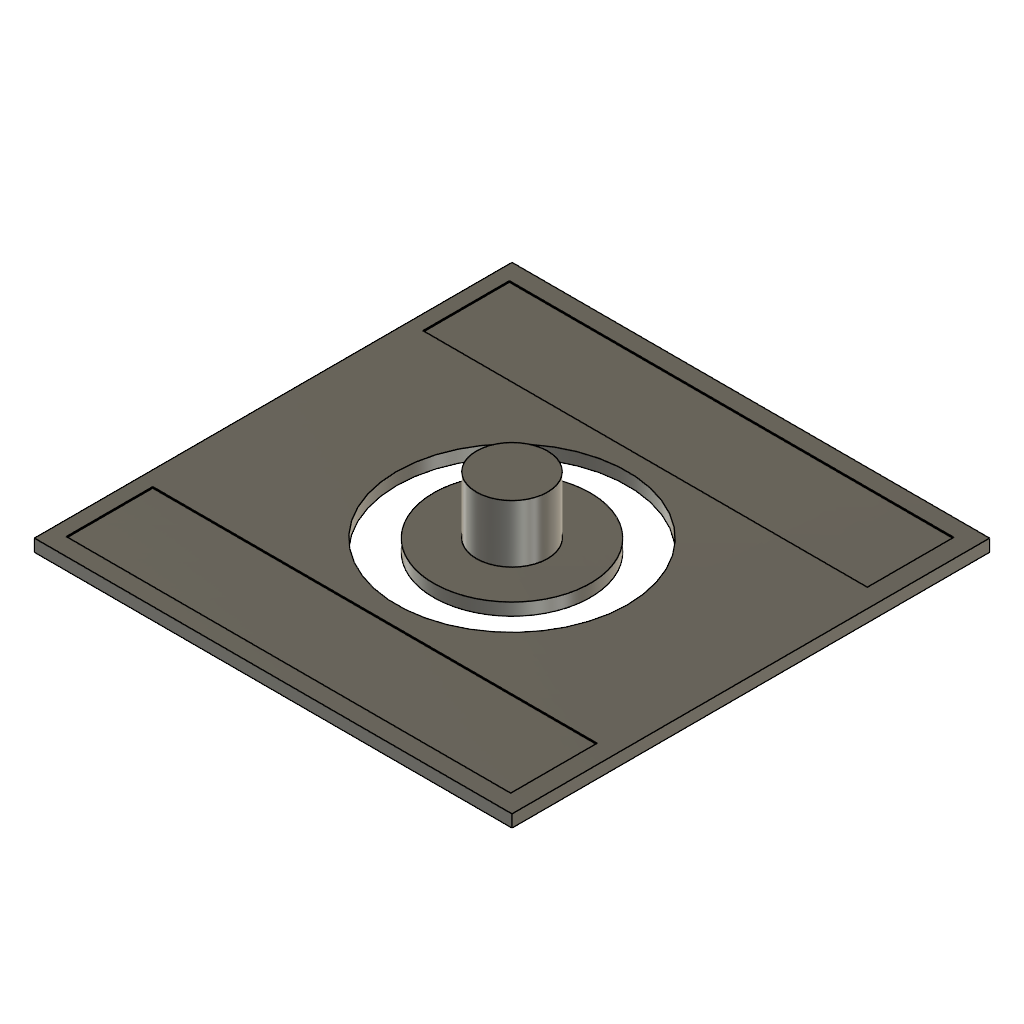
Power stencil (Autodesk Fusion 360 design; units mm, degrees)
Autodesk Fusion 360 part; units mm, degrees
sketch "Sketch1" plane through (0, 0, 0) normal (0, 0, 1) x (1, 0, 0)
  circle A0 centre (0, 0) radius 9.525
  dimension "d1" = 19.05
  constraint coincident A0.centre origin
  measures "d1" diameter of A0
extrude "Extrude1" add sketch "Sketch1" along normal blind 1.5 makes body 1
sketch "Sketch2" plane through (0, 0, 1.5) normal (0, 0, 1) x (-1, 0, 0)
  circle A0 centre (0, 0) radius 9.525
  line L0 (7, -5.7371) -> (-6, -5.7371)
  line L1 (-6, -5.7371) -> (-6, 5.2629)
  line L2 (-6, 5.2629) -> (7, 5.2629)
  line L3 (7, 5.2629) -> (7, -5.7371)
  dimension "d4" = 13
  dimension "d5" = 11
  constraint horizontal L0
  constraint vertical L1
  constraint horizontal L2
  constraint vertical L3
  measures "d4" distance of L0.start L0.end
  measures "d5" distance of L0.start L2.end
extrude "Extrude2" cut sketch "Sketch2" against normal blind 0.15 contours L0 L1 L2 L3 bodies 1
sketch "Sketch3" plane through (0, 0, 0) normal (0, 0, 1) x (1, 0, 0)
  line L0 (6, 5.7371) -> (6, -5.2629)
  line L1 (6, -5.2629) -> (-7, -5.2629)
  line L2 (-7, -5.2629) -> (-7, 5.7371)
  line L3 (-7, 5.7371) -> (6, 5.7371)
  circle A0 centre (0, 0) radius 9.525
  circle A1 centre (0, 0) radius 14.025
  line L4 (0, 14.025) -> (0, 29.025)
  line L5 (-14.025, 0) -> (-29.025, 0)
  line L6 (-29.025, 0) -> (-29.025, 29.025)
  line L7 (-29.025, 29.025) -> (29.025, 29.025)
  line L8 (29.025, 29.025) -> (29.025, -29.025)
  line L9 (29.025, -29.025) -> (-29.025, -29.025)
  line L10 (-29.025, -29.025) -> (-29.025, 29.025)
  dimension "d8" = 4.5
  dimension "d9" = 15
  dimension "d10" = 15
  dimension "d11" = 58.05
  dimension "d12" = 58.05
  constraint coincident A1 L4.start
  constraint perpendicular L3 L4
  constraint coincident A1 L5.start
  constraint perpendicular L2 L5
  constraint perpendicular L5 L6
  constraint horizontal L7
  constraint vertical L8
  constraint horizontal L9
  constraint vertical L10
  measures "d9" distance of L4.start L4.end
  measures "d10" distance of L5.start L5.end
  measures "d11" distance of L6.end L7.end
  measures "d12" distance of L6.end L9.end
extrude "Extrude3" add sketch "Sketch3" along normal blind 1.5 separate body contours A1 L4 L5 L7 L8 L9 L10 | A1 L4 L5 L6 L7 L10 makes body 2
sketch "Sketch4" plane through (0, 0, 1.5) normal (0, 0, 1) x (-1, 0, 0)
  circle A0 centre (0, 0) radius 14.025
  line L0 (29.025, 29.025) -> (-29.025, 29.025)
  line L1 (-29.025, 29.025) -> (-29.025, -29.025)
  line L2 (-29.025, -29.025) -> (29.025, -29.025)
  line L3 (29.025, -29.025) -> (29.025, 29.025)
  line L4 (27.2396, -26.9207) -> (-26.7604, -26.9207)
  line L5 (-26.7604, -26.9207) -> (-26.7604, -16.4207)
  line L6 (-26.7604, -16.4207) -> (27.2396, -16.4207)
  line L7 (27.2396, -16.4207) -> (27.2396, -26.9207)
  line L8 (0, 0) -> (-20.0107, 0)
  line L9 (-26.7604, 16.4207) -> (27.2396, 16.4207)
  line L10 (-26.7604, 26.9207) -> (-26.7604, 16.4207)
  line L11 (27.2396, 26.9207) -> (-26.7604, 26.9207)
  line L12 (27.2396, 16.4207) -> (27.2396, 26.9207)
  dimension "d15" = 54
  dimension "d16" = 10.5
  constraint horizontal L4
  constraint vertical L5
  constraint horizontal L6
  constraint vertical L7
  constraint coincident A0.centre L8.start
  constraint parallel L4 L8
  constraint symmetric L4.start L8 L11.start
  constraint symmetric L4.end L8 L10.start
  constraint symmetric L5.end L8 L9.start
  constraint symmetric L6.end L8 L9.end
  measures "d15" distance of L4.start L4.end
  measures "d16" distance of L4.start L6.end
extrude "Extrude4" cut sketch "Sketch4" against normal blind 0.15 contours L4 L5 L6 L7 | L9 L10 L11 L12 bodies 2
extrude "Extrude5" add 1 faces at (-2.6667, 2.0705, 1.35) along direction (0, 0, 1) blind 0.15 on bodies 1 bodies 1
sketch "Sketch5" plane through (0, 0, 1.5) normal (0, 0, 1) x (-1, 0, 0)
  circle A0 centre (0, 0) radius 9.525
  circle A1 centre (0, 0) radius 4.325
  dimension "d21" = 8.65
  constraint coincident A0.centre A1.centre
  measures "d21" diameter of A1
extrude "Extrude6" add sketch "Sketch5" along normal blind 7 contours A1 bodies 1
equation "d1 = 14.05 mm + 5 mm"
